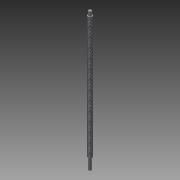
# Autodesk Inventor part: acmeScrew
Saved by Autodesk Inventor 2013 (Build 170138000, 138)
## iProperties
Created: 2012-12-05
Part Number: acmeScrew
Material: Generic
Document SubType Name: Modeling
Designer: Istvan
Density: 1 g/cm^3
Author: Istvan
Autodesk Inventor part; units mm, degrees
ref_plane "YZ Plane" through (0, 0, 0) normal (1, 0, 0) x (0, 1, 0)
ref_plane "XZ Plane" through (0, 0, 0) normal (0, 1, 0) x (-1, 0, 0)
ref_plane "XY Plane" through (0, 0, 0) normal (0, 0, 1) x (1, 0, 0)
sketch "Sketch1" plane through (0, 0, 0) normal (0, 1, 0) x (-1, 0, 0)
  circle A0 centre (0, 0) radius 4.7625
  dimension "d0" = 9.525
  constraints: 1 centre point, 1 coincident
  measures "d0" diameter of A0
extrude "Extrusion1" add sketch "Sketch1" along normal blind 304.8
thread "Thread1" size "3/8-12" class "2B" standard "Inch Tapping Threads" full length
sketch "Sketch2" plane through (0, 304.8, 0) normal (0, 1, 0) x (1, 0, 0)
  circle A0 centre (0, 0) radius 4.7625 projected
  arc A1 (1.7227, -2.667) -> (-1.7227, -2.667) centre (0, 0) ccw
  line L0 (-1.7227, -2.667) -> (1.7227, -2.667)
  dimension "d5" = 6.35
  dimension "d6" = 2.667
  constraints: 2 end point, 2 point on circle, 1 centre point, 1 coincident, 1 horizontal
  measures "d5" diameter of A1
  measures "d6" distance from line of L0 A0.centre
extrude "Extrusion2" cut sketch "Sketch2" against normal blind 9.525
sketch "Sketch3" plane through (0, 0, 0) normal (0, -1, 0) x (1, 0, 0)
  circle A0 centre (0, 0) radius 4.7625 projected
  circle A1 centre (0, 0) radius 3.175
  dimension "d9" = 6.35
  constraints: 1 centre point, 1 coincident
  measures "d9" diameter of A1
extrude "Extrusion3" cut sketch "Sketch3" against normal blind 25.4
body "Solid1"
